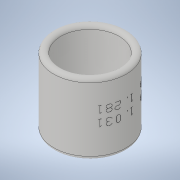
# Autodesk Inventor part: LargeFinderEyePieceCover
Saved by Autodesk Inventor 2020.2 (Build 242310000, 310)
## iProperties
Created: 2018-09-02
Part Number: LargeFinderEyePieceCover
Material: Generic
Document SubType Name: Modeling
Designer: steele
Density: 1 g/cm^3
Appearance: Default
Author: steele
Autodesk Inventor part; units mm, degrees
ref_plane "XZ Plane" through (0, 0, 0) normal (0, 1, 0) x (-1, 0, 0)
ref_plane "XY Plane" through (0, 0, 0) normal (0, 0, 1) x (1, 0, 0)
sketch "Sketch1" plane through (0, 0, 0) normal (0, 1, 0) x (-1, 0, 0)
  circle A0 centre (0, 0) radius 16.2735
  dimension "d0" = 32.547
  constraints: 1 centre point, 1 coincident
  measures "d0" diameter of A0
extrude "Extrusion1" add sketch "Sketch1" along normal blind 6.35
sketch "Sketch2" plane through (0, 6.35, 0) normal (0, 1, 0) x (1, 0, 0)
  circle A0 centre (0, 0) radius 16.2735
  circle A1 centre (0, 0) radius 13.0985
  dimension "d3" = 32.547
  dimension "d4" = 26.197
  constraints: 2 centre point, 2 coincident
  measures "d3" diameter of A0
  measures "d4" diameter of A1
extrude "Extrusion2" add sketch "Sketch2" along normal blind 25.4
ref_plane "Work Plane1" through (16.2735, 0, 0) normal (1, 0, 0) x (0, 1, 0)
sketch "Sketch3" plane through (16.2735, 0, 0) normal (1, 0, 0) x (0, 1, 0)
  line L0 (0, 16.2735) -> (31.75, 16.2735) construction
  line L1 (15.875, 16.2735) -> (15.875, -16.4842) construction
  line L2 (6.35, -13.0985) -> (31.75, -13.0985) construction
  line L3 (15.9058, -14.4393) -> (15.9058, -15.4553)
  line L4 (15.9058, -15.4553) -> (15.8391, -15.4553)
  line L5 (15.8391, -15.4553) -> (15.8391, -14.9807)
  line L6 (15.8391, -14.9807) -> (12.8604, -14.9807)
  line L7 (12.8604, -14.9807) -> (12.8604, -15.4553)
  line L8 (12.8604, -15.4553) -> (12.7936, -15.4553)
  line L9 (12.7936, -15.4553) -> (12.7936, -14.4393)
  line L10 (12.7936, -14.4393) -> (12.8604, -14.4393)
  line L11 (12.8604, -14.4393) -> (12.8604, -14.914)
  line L12 (12.8604, -14.914) -> (15.8391, -14.914)
  line L13 (15.8391, -14.914) -> (15.8391, -14.4393)
  line L14 (15.8391, -14.4393) -> (15.9058, -14.4393)
  line L15 (15.3798, -10.8269) -> (15.9058, -11.3554)
  line L16 (15.9058, -11.3554) -> (15.9058, -12.8922)
  line L17 (15.9058, -12.8922) -> (15.8391, -12.8922)
  line L18 (15.8391, -12.8922) -> (15.8391, -12.4176)
  line L19 (15.8391, -12.4176) -> (12.8604, -12.4176)
  line L20 (12.8604, -12.4176) -> (12.8604, -12.8922)
  line L21 (12.8604, -12.8922) -> (12.7936, -12.8922)
  line L22 (12.7936, -12.8922) -> (12.7936, -11.3554)
  line L23 (12.7936, -11.3554) -> (13.3222, -10.8269)
  line L24 (13.3222, -10.8269) -> (15.3798, -10.8269)
  line L25 (15.3542, -10.8936) -> (13.3478, -10.8936)
  line L26 (13.3478, -10.8936) -> (12.8604, -11.3836)
  line L27 (12.8604, -11.3836) -> (12.8604, -12.3509)
  line L28 (12.8604, -12.3509) -> (15.8391, -12.3509)
  line L29 (15.8391, -12.3509) -> (15.8391, -11.3836)
  line L30 (15.8391, -11.3836) -> (15.3542, -10.8936)
  line L31 (15.367, -9.7852) -> (15.367, -9.8545)
  line L32 (15.367, -9.8545) -> (14.859, -9.8545)
  line L33 (14.859, -9.8545) -> (14.859, -9.7852)
  line L34 (14.859, -9.7852) -> (15.367, -9.7852)
  line L35 (14.351, -9.7852) -> (14.351, -9.8545)
  line L36 (14.351, -9.8545) -> (13.8456, -9.8545)
  line L37 (13.8456, -9.8545) -> (13.8456, -9.7852)
  line L38 (13.8456, -9.7852) -> (14.351, -9.7852)
  line L39 (15.9058, -2.1421) -> (15.9058, -3.1581)
  line L40 (15.9058, -3.1581) -> (15.8391, -3.1581)
  line L41 (15.8391, -3.1581) -> (15.8391, -2.6835)
  line L42 (15.8391, -2.6835) -> (12.9065, -2.6835)
  line L43 (12.9065, -2.6835) -> (13.3607, -3.135)
  line L44 (13.3607, -3.135) -> (13.3093, -3.1838)
  line L45 (13.3093, -3.1838) -> (12.7936, -2.6655)
  line L46 (12.7936, -2.6655) -> (12.7936, -2.6168)
  line L47 (12.7936, -2.6168) -> (15.8391, -2.6168)
  line L48 (15.8391, -2.6168) -> (15.8391, -2.1421)
  line L49 (15.8391, -2.1421) -> (15.9058, -2.1421)
  line L50 (15.875, -0.572) -> (15.875, -0.6412)
  line L51 (15.875, -0.6412) -> (15.367, -0.6412)
  line L52 (15.367, -0.6412) -> (15.367, -0.572)
  line L53 (15.367, -0.572) -> (15.875, -0.572)
  line L54 (15.3798, 4.0206) -> (15.9058, 3.492)
  line L55 (15.9058, 3.492) -> (15.9058, 2.9584)
  line L56 (15.9058, 2.9584) -> (15.3798, 2.4299)
  line L57 (15.3798, 2.4299) -> (13.3222, 2.4299)
  line L58 (13.3222, 2.4299) -> (12.7936, 2.9584)
  line L59 (12.7936, 2.9584) -> (12.7936, 3.492)
  line L60 (12.7936, 3.492) -> (13.3222, 4.0206)
  line L61 (13.3222, 4.0206) -> (15.3798, 4.0206)
  line L62 (15.3542, 3.9513) -> (13.3478, 3.9513)
  line L63 (13.3478, 3.9513) -> (12.8604, 3.4664)
  line L64 (12.8604, 3.4664) -> (12.8604, 2.984)
  line L65 (12.8604, 2.984) -> (13.3478, 2.4991)
  line L66 (13.3478, 2.4991) -> (15.3542, 2.4991)
  line L67 (15.3542, 2.4991) -> (15.8391, 2.984)
  line L68 (15.8391, 2.984) -> (15.8391, 3.4664)
  line L69 (15.8391, 3.4664) -> (15.3542, 3.9513)
  line L70 (15.3798, 7.5997) -> (15.9058, 7.0711)
  line L71 (15.9058, 7.0711) -> (15.9058, 6.0295)
  line L72 (15.9058, 6.0295) -> (15.3901, 5.5086)
  line L73 (15.3901, 5.5086) -> (15.3413, 5.56)
  line L74 (15.3413, 5.56) -> (15.8391, 6.0551)
  line L75 (15.8391, 6.0551) -> (15.8391, 7.0429)
  line L76 (15.8391, 7.0429) -> (15.3542, 7.533)
  line L77 (15.3542, 7.533) -> (14.8693, 7.533)
  line L78 (14.8693, 7.533) -> (14.3844, 7.0429)
  line L79 (14.3844, 7.0429) -> (14.3844, 6.5503)
  line L80 (14.3844, 6.5503) -> (14.3176, 6.5503)
  line L81 (14.3176, 6.5503) -> (14.3176, 7.0429)
  line L82 (14.3176, 7.0429) -> (13.8302, 7.533)
  line L83 (13.8302, 7.533) -> (13.3478, 7.533)
  line L84 (13.3478, 7.533) -> (12.8604, 7.0429)
  line L85 (12.8604, 7.0429) -> (12.8604, 6.0551)
  line L86 (12.8604, 6.0551) -> (13.3607, 5.56)
  line L87 (13.3607, 5.56) -> (13.3093, 5.5086)
  line L88 (13.3093, 5.5086) -> (12.7936, 6.0295)
  line L89 (12.7936, 6.0295) -> (12.7936, 7.0711)
  line L90 (12.7936, 7.0711) -> (13.3222, 7.5997)
  line L91 (13.3222, 7.5997) -> (13.8558, 7.5997)
  line L92 (13.8558, 7.5997) -> (14.3484, 7.1045)
  line L93 (14.3484, 7.1045) -> (14.8462, 7.5997)
  line L94 (14.8462, 7.5997) -> (15.3798, 7.5997)
  line L95 (15.9058, 10.1422) -> (15.9058, 9.1262)
  line L96 (15.9058, 9.1262) -> (15.8391, 9.1262)
  line L97 (15.8391, 9.1262) -> (15.8391, 9.6009)
  line L98 (15.8391, 9.6009) -> (12.9065, 9.6009)
  line L99 (12.9065, 9.6009) -> (13.3607, 9.1493)
  line L100 (13.3607, 9.1493) -> (13.3093, 9.1006)
  line L101 (13.3093, 9.1006) -> (12.7936, 9.6188)
  line L102 (12.7936, 9.6188) -> (12.7936, 9.6676)
  line L103 (12.7936, 9.6676) -> (15.8391, 9.6676)
  line L104 (15.8391, 9.6676) -> (15.8391, 10.1422)
  line L105 (15.8391, 10.1422) -> (15.9058, 10.1422)
  line L106 (21.0987, -13.898) -> (21.0987, -15.9967)
  line L107 (21.0987, -15.9967) -> (17.9865, -15.9967)
  line L108 (17.9865, -15.9967) -> (17.9865, -13.898)
  line L109 (17.9865, -13.898) -> (21.0987, -13.898)
  line L110 (21.0319, -13.9647) -> (18.0532, -13.9647)
  line L111 (18.0532, -13.9647) -> (18.0532, -15.9274)
  line L112 (18.0532, -15.9274) -> (21.0319, -15.9274)
  line L113 (21.0319, -15.9274) -> (21.0319, -13.9647)
  line L114 (20.5727, -10.8269) -> (21.0987, -11.3554)
  line L115 (21.0987, -11.3554) -> (21.0987, -12.8922)
  line L116 (21.0987, -12.8922) -> (21.0319, -12.8922)
  line L117 (21.0319, -12.8922) -> (21.0319, -12.4176)
  line L118 (21.0319, -12.4176) -> (18.0532, -12.4176)
  line L119 (18.0532, -12.4176) -> (18.0532, -12.8922)
  line L120 (18.0532, -12.8922) -> (17.9865, -12.8922)
  line L121 (17.9865, -12.8922) -> (17.9865, -11.3554)
  line L122 (17.9865, -11.3554) -> (18.515, -10.8269)
  line L123 (18.515, -10.8269) -> (20.5727, -10.8269)
  line L124 (20.547, -10.8936) -> (18.5407, -10.8936)
  line L125 (18.5407, -10.8936) -> (18.0532, -11.3836)
  line L126 (18.0532, -11.3836) -> (18.0532, -12.3509)
  line L127 (18.0532, -12.3509) -> (21.0319, -12.3509)
  line L128 (21.0319, -12.3509) -> (21.0319, -11.3836)
  line L129 (21.0319, -11.3836) -> (20.547, -10.8936)
  line L130 (20.5599, -9.7852) -> (20.5599, -9.8545)
  line L131 (20.5599, -9.8545) -> (20.0519, -9.8545)
  line L132 (20.0519, -9.8545) -> (20.0519, -9.7852)
  line L133 (20.0519, -9.7852) -> (20.5599, -9.7852)
  line L134 (19.5439, -9.7852) -> (19.5439, -9.8545)
  line L135 (19.5439, -9.8545) -> (19.0384, -9.8545)
  line L136 (19.0384, -9.8545) -> (19.0384, -9.7852)
  line L137 (19.0384, -9.7852) -> (19.5439, -9.7852)
  line L138 (21.0987, -2.1421) -> (21.0987, -3.1581)
  line L139 (21.0987, -3.1581) -> (21.0319, -3.1581)
  line L140 (21.0319, -3.1581) -> (21.0319, -2.6835)
  line L141 (21.0319, -2.6835) -> (18.0994, -2.6835)
  line L142 (18.0994, -2.6835) -> (18.5535, -3.135)
  line L143 (18.5535, -3.135) -> (18.5022, -3.1838)
  line L144 (18.5022, -3.1838) -> (17.9865, -2.6655)
  line L145 (17.9865, -2.6655) -> (17.9865, -2.6168)
  line L146 (17.9865, -2.6168) -> (21.0319, -2.6168)
  line L147 (21.0319, -2.6168) -> (21.0319, -2.1421)
  line L148 (21.0319, -2.1421) -> (21.0987, -2.1421)
  line L149 (21.0679, -0.572) -> (21.0679, -0.6412)
  line L150 (21.0679, -0.6412) -> (20.5599, -0.6412)
  line L151 (20.5599, -0.6412) -> (20.5599, -0.572)
  line L152 (20.5599, -0.572) -> (21.0679, -0.572)
  line L153 (19.0487, 4.5286) -> (19.5772, 4)
  line L154 (19.5772, 4) -> (19.5772, 2.984)
  line L155 (19.5772, 2.984) -> (20.0621, 2.4991)
  line L156 (20.0621, 2.4991) -> (21.0319, 2.4991)
  line L157 (21.0319, 2.4991) -> (21.0319, 4.4926)
  line L158 (21.0319, 4.4926) -> (21.0987, 4.4926)
  line L159 (21.0987, 4.4926) -> (21.0987, 2.4299)
  line L160 (21.0987, 2.4299) -> (20.039, 2.4299)
  line L161 (20.039, 2.4299) -> (19.5105, 2.9584)
  line L162 (19.5105, 2.9584) -> (19.5105, 3.9718)
  line L163 (19.5105, 3.9718) -> (19.023, 4.4619)
  line L164 (19.023, 4.4619) -> (18.5407, 4.4619)
  line L165 (18.5407, 4.4619) -> (18.0532, 3.9718)
  line L166 (18.0532, 3.9718) -> (18.0532, 2.984)
  line L167 (18.0532, 2.984) -> (18.5535, 2.4889)
  line L168 (18.5535, 2.4889) -> (18.5022, 2.4376)
  line L169 (18.5022, 2.4376) -> (17.9865, 2.9584)
  line L170 (17.9865, 2.9584) -> (17.9865, 4)
  line L171 (17.9865, 4) -> (18.515, 4.5286)
  line L172 (18.515, 4.5286) -> (19.0487, 4.5286)
  line L173 (20.5727, 7.5997) -> (21.0987, 7.0711)
  line L174 (21.0987, 7.0711) -> (21.0987, 6.0295)
  line L175 (21.0987, 6.0295) -> (20.5727, 5.501)
  line L176 (20.5727, 5.501) -> (20.039, 5.501)
  line L177 (20.039, 5.501) -> (19.5413, 5.9936)
  line L178 (19.5413, 5.9936) -> (19.0487, 5.501)
  line L179 (19.0487, 5.501) -> (18.515, 5.501)
  line L180 (18.515, 5.501) -> (17.9865, 6.0295)
  line L181 (17.9865, 6.0295) -> (17.9865, 7.0711)
  line L182 (17.9865, 7.0711) -> (18.515, 7.5997)
  line L183 (18.515, 7.5997) -> (19.0487, 7.5997)
  line L184 (19.0487, 7.5997) -> (19.5413, 7.1045)
  line L185 (19.5413, 7.1045) -> (20.039, 7.5997)
  line L186 (20.039, 7.5997) -> (20.5727, 7.5997)
  line L187 (19.023, 7.533) -> (18.5407, 7.533)
  line L188 (18.5407, 7.533) -> (18.0532, 7.0429)
  line L189 (18.0532, 7.0429) -> (18.0532, 6.0551)
  line L190 (18.0532, 6.0551) -> (18.5407, 5.5702)
  line L191 (18.5407, 5.5702) -> (19.023, 5.5702)
  line L192 (19.023, 5.5702) -> (19.5105, 6.0551)
  line L193 (19.5105, 6.0551) -> (19.5105, 7.0429)
  line L194 (19.5105, 7.0429) -> (19.023, 7.533)
  line L195 (20.547, 7.533) -> (20.0647, 7.533)
  line L196 (20.0647, 7.533) -> (19.5772, 7.0429)
  line L197 (19.5772, 7.0429) -> (19.5772, 6.0551)
  line L198 (19.5772, 6.0551) -> (20.0647, 5.5702)
  line L199 (20.0647, 5.5702) -> (20.547, 5.5702)
  line L200 (20.547, 5.5702) -> (21.0319, 6.0551)
  line L201 (21.0319, 6.0551) -> (21.0319, 7.0429)
  line L202 (21.0319, 7.0429) -> (20.547, 7.533)
  line L203 (21.0987, 10.1422) -> (21.0987, 9.1262)
  line L204 (21.0987, 9.1262) -> (21.0319, 9.1262)
  line L205 (21.0319, 9.1262) -> (21.0319, 9.6009)
  line L206 (21.0319, 9.6009) -> (18.0994, 9.6009)
  line L207 (18.0994, 9.6009) -> (18.5535, 9.1493)
  line L208 (18.5535, 9.1493) -> (18.5022, 9.1006)
  line L209 (18.5022, 9.1006) -> (17.9865, 9.6188)
  line L210 (17.9865, 9.6188) -> (17.9865, 9.6676)
  line L211 (17.9865, 9.6676) -> (21.0319, 9.6676)
  line L212 (21.0319, 9.6676) -> (21.0319, 10.1422)
  line L213 (21.0319, 10.1422) -> (21.0987, 10.1422)
  point P0 (0, 0)
  constraints: 2 end point, 1 midpoint, 1 perpendicular, 1 vertical
emboss "Emboss1" sketch "Sketch3" operation cut depth 2.54 direction (1, 0, 0) wrap yes faces at (-16.0628, 12.7, -2.6105)
fillet "Fillet1" radius 1.5875 1 edges at (16.2735, 0, 0)
fillet "Fillet2" radius 1.5875 2 edges at (-13.0985, 31.75, 0) (-16.2735, 31.75, 0)
equation "\"d0\" = coverOD"
equation "\"d1\" = wallThickness"
equation "\"d3\" = coverOD"
equation "\"d4\" = eypPieceCoverID"
equation "\"wallThickness\" = 6.35"
equation "\"coverOD\" = eypPieceCoverID + wallThickness"
equation "\"eypPieceCoverID\" = 26.197"
body "Solid1"
